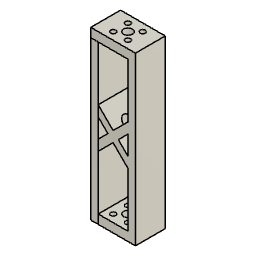
大臂 v4 (Autodesk Fusion 360 design; units mm, degrees)
Autodesk Fusion 360 part; units mm, degrees
sketch "草图1" plane through (0, 0, 0) normal (0, 0, 1) x (1, 0, 0)
  line L0 (15, -10) -> (-15, -10)
  line L1 (-15, -10) -> (-15, 10)
  line L2 (-15, 10) -> (15, 10)
  line L3 (15, 10) -> (15, -10)
  line L4 (15, -10) -> (-15, 10) construction
  line L5 (-15, -10) -> (15, 10) construction
  line L6 (0, 0) -> (19, 0) construction
  line L7 (0, 0) -> (9.0277, 9.0277) construction
  circle A0 centre (0, 0) radius 7 construction
  circle A1 centre (4.9497, 4.9497) radius 1.75
  circle A2 centre (-4.9497, 4.9497) radius 1.75
  circle A3 centre (-4.9497, -4.9497) radius 1.75
  circle A4 centre (4.9497, -4.9497) radius 1.75
  circle A5 centre (0, 0) radius 3
  dimension "d1" = 20
  dimension "d2" = 30
  dimension "d3" = 45
  dimension "d4" = 14
  dimension "d5" = 3.5
  dimension "d7" = 360
  dimension "d8" = 6
  constraint horizontal L0
  constraint perpendicular L0 L1
  constraint parallel L0 L2
  constraint parallel L1 L3
  constraint coincident L4 L6.start
  constraint coincident L5 L6.start
  constraint coincident L6.start L7.start
  constraint horizontal L6
  constraint coincident A0 A1.centre
  constraint coincident L7 A1.centre
  measures "d1" distance of L0.end L1.end
  measures "d2" distance of L1.end L2.end
  measures "d3" angle of L6 L7
  measures "d4" diameter of A0
  measures "d5" diameter of A1
  measures "d8" diameter of A5
  measures "d12" distance of A1.centre
extrude "拉伸1" add sketch "草图1" along normal blind 6 makes body 1
sketch "草图2" plane through (0, 0, 0) normal (0, 0, -1) x (1, 0, 0)
  circle A0 centre (0, 0) radius 3
  circle A1 centre (4.9497, -4.9497) radius 1.75
  circle A2 centre (-4.9497, 4.9497) radius 1.75
  circle A3 centre (4.9497, 4.9497) radius 1.75
  circle A4 centre (-4.9497, -4.9497) radius 1.75
  line L0 (-15, -10) -> (15, -10)
  line L1 (15, -10) -> (15, 10)
  line L2 (15, 10) -> (-15, 10)
  line L3 (-15, 10) -> (-15, -10)
  line L4 (15, -10) -> (10, -10)
  line L5 (10, -10) -> (10, 10)
  line L6 (10, 10) -> (15, 10)
  line L7 (15, 10) -> (15, -10)
  line L8 (-15, -10) -> (-10, -10)
  line L9 (-10, -10) -> (-10, 10)
  line L10 (-10, 10) -> (-15, 10)
  line L11 (-15, 10) -> (-15, -10)
  dimension "d11" = 5
  dimension "d12" = 5
  constraint horizontal L4
  constraint vertical L5
  constraint horizontal L6
  constraint vertical L7
  constraint coincident L2 L5.end
  constraint coincident L0.end L1.start
  constraint horizontal L8
  constraint vertical L9
  constraint horizontal L10
  constraint vertical L11
  constraint coincident L2 L9.end
  constraint coincident L0.start L3.end
  measures "d11" distance of L0.end L4.end
  measures "d12" distance of L0.start L8.end
extrude "拉伸2" add sketch "草图2" along normal blind 100 contours L0 L2 L3 L8 L9 L10 L11 | L0 L1 L2 L4 L5 L6 L7 bodies 1
sketch "草图3" plane through (0, 0, -100) normal (0, 0, -1) x (1, 0, 0)
  line L0 (-15, 10) -> (-15, -10)
  line L1 (-15, -10) -> (-10, -10)
  line L2 (-10, -10) -> (-10, 10)
  line L3 (-10, 10) -> (-15, 10)
  line L4 (-10, 10) -> (-10, -10)
  line L5 (-10, -10) -> (10, -10)
  line L6 (10, -10) -> (10, 10)
  line L7 (10, 10) -> (-10, 10)
  circle A0 centre (-4.9497, -4.9497) radius 1.75
  circle A1 centre (4.9497, 4.9497) radius 1.75
  circle A2 centre (-4.9497, 4.9497) radius 1.75
  circle A3 centre (4.9497, -4.9497) radius 1.75
  circle A4 centre (0, 0) radius 3
  line L8 (15, 10) -> (10, 10)
  line L9 (10, 10) -> (10, -10)
  line L10 (10, -10) -> (15, -10)
  line L11 (15, -10) -> (15, 10)
extrude "拉伸3" add sketch "草图3" along normal blind 6 bodies 1
sketch "草图4" plane through (0, 10, 0) normal (0, 1, 0) x (-1, 0, 0)
  line L0 (15, -106) -> (15, 6)
  line L1 (15, 6) -> (-15, 6)
  line L2 (-15, 6) -> (-15, -106)
  line L3 (-15, -106) -> (15, -106)
  line L4 (10, -100) -> (-10, -100)
  line L5 (-10, -100) -> (-10, 0)
  line L6 (-10, 0) -> (10, 0)
  line L7 (10, 0) -> (10, -100)
  line L8 (47.9011, -50) -> (-70, -50)
  line L9 (0, -112.7701) -> (0, 40) construction
  line L10 (-10, -63.5355) -> (-13.5355, -60)
  line L11 (-13.5355, -60) -> (10, -36.4645)
  line L12 (10, -36.4645) -> (13.5355, -40)
  line L13 (13.5355, -40) -> (-10, -63.5355)
  line L14 (-10, -63.5355) -> (10, -36.4645)
  line L15 (13.5355, -40) -> (-13.5355, -60)
  line L16 (-10, -36.4645) -> (-13.5355, -40)
  line L17 (13.5355, -60) -> (-10, -36.4645)
  line L18 (-13.5355, -40) -> (10, -63.5355)
  line L19 (10, -63.5355) -> (13.5355, -60)
  line L20 (-10, -36.4645) -> (10, -63.5355)
  line L21 (13.5355, -60) -> (-13.5355, -40)
  point P0 (0, -50)
  dimension "d17" = 45
  dimension "d18" = 5
  constraint perpendicular L5 L8
  constraint symmetric L4 L6 L8
  constraint vertical L9
  constraint perpendicular L10 L11
  constraint parallel L10 L12
  constraint parallel L11 L13
  constraint coincident L5 L10.start
  constraint midpoint L15 P0
  constraint coincident L8 P0
  constraint coincident L9 P0
  constraint symmetric L8 L10.start L16.start
  constraint symmetric L8 L10.end L16.end
  constraint symmetric L8 L11.end L18.end
  constraint symmetric L8 L12.end L17.start
  measures "d17" angle of L8 L11
  measures "d18" distance of L10.start L10.end
extrude "拉伸4" add sketch "草图4" against normal blind 20 contours L7 L13 L15 L17 | L7 L13 L17 L21 | L8 L13 L21 | L8 L15 L17 | L7 L14 L15 L17 | L7 L13 L20 L21 | L8 L15 L18 | L13 L14 L18 L20 | L11 L14 L17 L20 | L14 L15 L17 | L14 L15 L18 | L11 L20 L21 | L13 L20 L21 | L8 L11 L21 | L5 L11 L15 L18 | L5 L11 L18 L21 | L11 L14 L17 | L13 L18 L20 | L13 L14 L18 | L5 L14 L15 L18 | L11 L17 L20 | L5 L11 L20 L21 bodies 1
sketch "草图5" plane through (0, 0, -106) normal (0, 0, -1) x (1, 0, 0)
  circle A0 centre (4.9497, -4.9497) radius 1.75
  circle A1 centre (4.9497, 4.9497) radius 1.75
  circle A2 centre (-4.9497, 4.9497) radius 1.75
  circle A3 centre (0, 0) radius 3
  circle A4 centre (-4.9497, -4.9497) radius 1.75
  line L0 (15, -10) -> (15, 10)
  line L1 (15, 10) -> (-10, 10)
  line L2 (-10, 10) -> (-15, 10)
  line L3 (-15, 10) -> (-15, -10)
  line L4 (-15, -10) -> (15, -10)
  circle A5 centre (0, 0) radius 3
extrude "拉伸5" cut sketch "草图5" against normal blind 112 contours A3 A5 bodies 1
copy_body "实体->零部件1" bodies 1 removing the originals makes body 2 in component "大臂"
component "大臂" placed x (1, 0, 0) y (0, 1, 0) z (0, 0, 1) at (0, 0, 0)
named bodies: "大臂"
